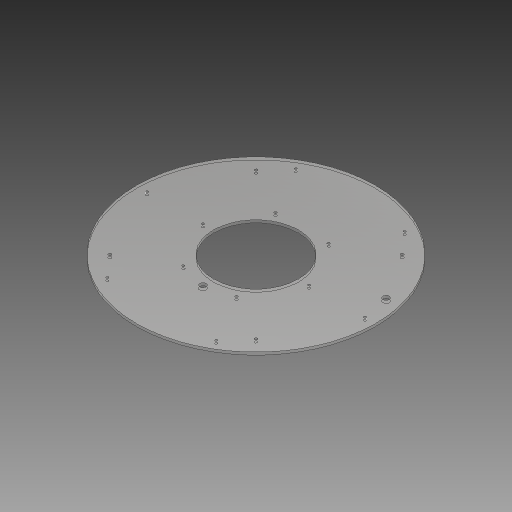
# Autodesk Inventor part: Primary
Saved by Autodesk Inventor 2019 (Build 230136000, 136)
## iProperties
Created: 2018-04-27
Part Number: Primary
Material: Polycarbonate, Clear
Document SubType Name: Modeling
Designer: Phil Erle
Density: 1.2 g/cm^3
Appearance: Polycarbonate - Clear
Author: Phil Erle
Autodesk Inventor part; units mm, degrees
ref_plane "YZ Plane" through (0, 0, 0) normal (1, 0, 0) x (0, 1, 0)
ref_plane "XZ Plane" through (0, 0, 0) normal (0, 1, 0) x (-1, 0, 0)
ref_plane "XY Plane" through (0, 0, 0) normal (0, 0, 1) x (1, 0, 0)
sketch "Sketch1" plane through (0, 0, 0) normal (0, 0, 1) x (1, 0, 0)
  circle A0 centre (0, 0) radius 80
  circle A1 centre (0, 0) radius 225
  dimension "d0" = 160
  dimension "d1" = 450
  constraints: 2 centre point, 2 coincident
  measures "d0" diameter of A0
  measures "d1" diameter of A1
extrude "Extrusion1" add sketch "Sketch1" along normal blind 5
sketch "Sketch2" plane through (0, 0, 5) normal (0, 0, 1) x (1, 0, 0)
  line L0 (-205, 0) -> (-100, 0) construction
  point P0 (0, 0)
  point P1 (-102.5, -177.5352)
  point P2 (-50, -86.6025)
  point P3 (102.5, -177.5352)
  point P4 (50, -86.6025)
  point P5 (205, 0)
  point P6 (100, 0)
  point P7 (102.5, 177.5352)
  point P8 (50, 86.6025)
  point P9 (-102.5, 177.5352)
  point P10 (-50, 86.6025)
  dimension "d4" = 100
  dimension "d5" = 205
  dimension "d8" = 360
  constraints: 2 coincident, 2 end point, 1 horizontal, 1 horizontal alignment, 13 other
  measures "d4" distance of point (0, 0) L0.end
  measures "d5" distance of point (0, 0) L0.start
hole "Hole1" at (-205, 0, 5) at (-100, 0, 5) at (-102.5, -177.5352, 5) at (-50, -86.6025, 5) at (102.5, -177.5352, 5) at (50, -86.6025, 5) at (205, 0, 5) at (100, 0, 5) at (102.5, 177.5352, 5) at (50, 86.6025, 5) at (-102.5, 177.5352, 5) at (-50, 86.6025, 5) direction (0, 0, -1) diameter 4.5 depth 8 tip angle 118 clearance for "Countersunk Flat Head Screw DIN EN ISO 2009" size "M4" standard "DIN"
sketch "Sketch3" plane through (0, 0, 5) normal (0, 0, 1) x (1, 0, 0)
  line L0 (-137.5, -137.5) -> (137.5, -137.5) construction
  line L1 (137.5, -137.5) -> (137.5, 137.5) construction
  line L2 (137.5, 137.5) -> (-137.5, 137.5) construction
  line L3 (-137.5, 137.5) -> (-137.5, -137.5) construction
  line L4 (-137.5, -137.5) -> (137.5, 137.5) construction
  line L5 (137.5, -137.5) -> (-137.5, 137.5) construction
  point P0 (0, 0)
  dimension "d17" = 275
  dimension "d18" = 275
  constraints: 12 end point, 4 coincident, 2 midpoint, 2 parallel, 1 horizontal, 1 perpendicular
  measures "d17" distance of L2.end L1.end
  measures "d18" distance of L1.end L0.end
hole "Hole2" at (-137.5, 137.5, 5) at (137.5, -137.5, 5) at (-137.5, -137.5, 5) at (137.5, 137.5, 5) direction (0, 0, -1) diameter 5.5 depth 8 tip angle 118 clearance for "Countersunk Flat Head Screw DIN EN ISO 2009" size "M5" standard "DIN"
sketch "Sketch4" plane through (0, 0, 5) normal (0, 0, 1) x (1, 0, 0)
  line L0 (0, 0) -> (193.1852, 51.7638) construction
  line L1 (0, 0) -> (-138.753, 0) construction
  point P0 (0, -100)
  dimension "d26" = 100
  dimension "d38" = 200
  dimension "d39" = 165
  constraints: 4 end point, 1 coincident, 1 horizontal, 1 vertical alignment
  measures "d26" distance of L0.start point (0, -100)
  measures "d38" distance of L0.start L0.end
  measures "d39" angle of L0 L1
hole "Hole3" at (0, -100, 5) at (193.1852, 51.7638, 5) direction (0, 0, -1) diameter 12 depth 8 tip angle 118
body "Solid1"
